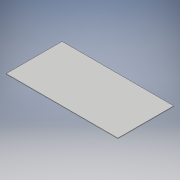
# Autodesk Inventor part: Foor
Saved by Autodesk Inventor 2018 (Build 220112000, 112)
## iProperties
Created: 2019-05-10
Part Number: Foor
Material: Generic
Document SubType Name: Modeling
Designer: 10043883
Density: 1 g/cm^3
Appearance: Default
Author: 10043883
Autodesk Inventor part; units mm, degrees
ref_plane "YZ Plane" through (0, 0, 0) normal (1, 0, 0) x (0, 1, 0)
ref_plane "XZ Plane" through (0, 0, 0) normal (0, 1, 0) x (-1, 0, 0)
ref_plane "XY Plane" through (0, 0, 0) normal (0, 0, 1) x (1, 0, 0)
sketch "Sketch1" plane through (0, 0, 0) normal (0, 1, 0) x (-1, 0, 0)
  line L0 (3048, 1524) -> (-3048, 1524)
  line L1 (-3048, 1524) -> (-3048, -1524)
  line L2 (-3048, -1524) -> (3048, -1524)
  line L3 (3048, -1524) -> (3048, 1524)
  line L4 (3048, 1524) -> (-3048, -1524) construction
  line L5 (-3048, 1524) -> (3048, -1524) construction
  point P0 (0, 0)
  dimension "d0" = 6096
  dimension "d1" = 3048
  constraints: 12 end point, 2 midpoint, 2 parallel, 1 horizontal, 1 perpendicular
  measures "d0" distance of L2.end L1.end
  measures "d1" distance of L1.end L0.end
extrude "Extrusion1" add sketch "Sketch1" along normal blind 25.4
body "Solid1"
